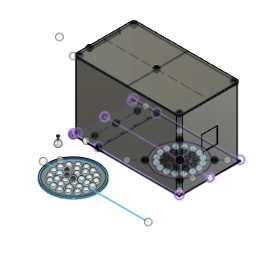
smallAmp v14 (Autodesk Fusion 360 design; units mm, degrees)
Autodesk Fusion 360 part; units mm, degrees
note: some values were not read from the file. Set by a fixed rule: which sketch regions a step uses.
sketch "Base" plane through (0, 0, 0) normal (0, 1, 0) x (1, 0, 0) in component "Top"
  line L0 (0, 0) -> (140, 0)
  line L1 (140, 0) -> (140, 80)
  line L2 (140, 80) -> (0, 80)
  line L3 (0, 80) -> (0, 0)
  dimension "d6" = 140
  dimension "d7" = 80
  constraint horizontal L0
  constraint vertical L1
  constraint horizontal L2
  constraint vertical L3
  constraint coincident L0.start L3.end
  measures "d6" distance of L0.start L0.end
  measures "d7" distance of L0.start L2.end
extrude "Extrude1" add sketch "Base" along normal blind 90 makes body 1 in component "Top"
fillet "Fillet1" radius 4 4 edges at (140, 45, 0) (0, 45, 0) (140, 45, -80) (0, 45, -80) on bodies 1 in component "Top"
shell "Shell1" thickness 1.5 removed faces 1 at (92, 90, -26.6667) on bodies 1 in component "Top"
sketch "Knob" plane through (1.5, 0, 0) normal (1, 0, 0) x (0, 0, -1) in component "Top"
  line L0 (76, 1.5) -> (76, 90)
  line L1 (76, 90) -> (4, 90)
  line L2 (4, 90) -> (4, 1.5)
  line L3 (4, 1.5) -> (76, 1.5)
  line L4 (20, 90) -> (60, 90)
  line L5 (60, 90) -> (60, 87)
  line L6 (60, 87) -> (20, 87)
  line L7 (20, 87) -> (20, 90)
  line L8 (40, 90) -> (40, 87) construction
  dimension "d12" = 40
  dimension "d13" = 3
  constraint horizontal L4
  constraint vertical L5
  constraint horizontal L6
  constraint vertical L7
  constraint coincident L1 L4.start
  constraint midpoint L1 L8.start
  constraint midpoint L6 L8.end
  constraint vertical L8
  measures "d12" distance of L5.end L6.end
  measures "d13" distance of L4.end L5.end
extrude "Extrude2" add sketch "Knob" along normal blind 6 draft -45 contours L1 L4 L5 L6 L7 bodies 1 in component "Top"
ref_plane "WorkPlane2" through (70, 45, -40) normal (-1, 0, 0) x (0, 0, 1) in component "Top"
mirror "Mirror1" about plane through (70, 45, -40) normal (-1, 0, 0) of "Extrude2" in component "Top"
sketch "Top" plane through (0, 90, 0) normal (0, 1, 0) x (-1, 0, 0) in component "Base"
  line L0 (-140, -4) -> (-140, -76)
  arc A0 (-140, -76) -> (-136, -80) centre (-136, -76) ccw
  line L1 (-136, -80) -> (-4, -80)
  arc A1 (-4, -80) -> (0, -76) centre (-4, -76) ccw
  line L2 (0, -76) -> (0, -4)
  arc A2 (0, -4) -> (-4, 0) centre (-4, -4) ccw
  line L3 (-4, 0) -> (-136, 0)
  arc A3 (-136, 0) -> (-140, -4) centre (-136, -4) ccw
  line L4 (-138.5, -20) -> (-138.5, -4)
  arc A4 (-136, -1.5) -> (-138.5, -4) centre (-136, -4) ccw
  line L5 (-136, -1.5) -> (-4, -1.5)
  arc A5 (-1.5, -4) -> (-4, -1.5) centre (-4, -4) ccw
  line L6 (-1.5, -4) -> (-1.5, -20)
  line L7 (-1.5, -20) -> (-1.5, -60)
  line L8 (-1.5, -60) -> (-1.5, -76)
  arc A6 (-4, -78.5) -> (-1.5, -76) centre (-4, -76) ccw
  line L9 (-4, -78.5) -> (-136, -78.5)
  arc A7 (-138.5, -76) -> (-136, -78.5) centre (-136, -76) ccw
  line L10 (-138.5, -76) -> (-138.5, -60)
  line L11 (-138.5, -60) -> (-138.5, -20)
  line L12 (0, -40) -> (-140, -40) construction
  line L13 (-70, -80) -> (-70, 0)
  point P0 (30.9232, -12.6835)
  point P1 (-70, -40)
  constraint midpoint L2 L12.start
  constraint midpoint L0 L12.end
  constraint midpoint L1 L13.start
  constraint midpoint L3 L13.end
  constraint midpoint L13 P1
extrude "Extrude1'" add sketch "Top" along normal blind 1.5 separate body makes body 2 in component "Base"
sketch "Lip" plane through (0, 90, 0) normal (0, -1, 0) x (1, 0, 0) in component "Base"
  arc A0 (140, -4) -> (136, 0) centre (136, -4) ccw
  line L0 (136, 0) -> (4, 0)
  arc A1 (4, 0) -> (0, -4) centre (4, -4) ccw
  line L1 (0, -4) -> (0, -76)
  arc A2 (0, -76) -> (4, -80) centre (4, -76) ccw
  line L2 (4, -80) -> (136, -80)
  arc A3 (136, -80) -> (140, -76) centre (136, -76) ccw
  line L3 (140, -76) -> (140, -4)
  line L4 (138.3, -76) -> (138.3, -4)
  arc A4 (138.3, -4) -> (136, -1.7) centre (136, -4) ccw
  line L5 (136, -1.7) -> (4, -1.7)
  arc A5 (4, -1.7) -> (1.7, -4) centre (4, -4) ccw
  line L6 (1.7, -4) -> (1.7, -76)
  arc A6 (1.7, -76) -> (4, -78.3) centre (4, -76) ccw
  line L7 (4, -78.3) -> (136, -78.3)
  arc A7 (136, -78.3) -> (138.3, -76) centre (136, -76) ccw
  dimension "d19" = 1.7
extrude "Extrude2'" add sketch "Lip" along normal blind 3 contours L4 A4 L5 A5 L6 A6 L7 A7 bodies 2 in component "Base"
extrude "Extrude3" cut sketch "Knob" along normal blind 3 draft -45 from surface at 0.2 contours L1 L4 L5 L6 L7 bodies 2 in component "Base"
mirror "Mirror1'" about plane through (70, 45, -40) normal (-1, 0, 0) of "Extrude3" in component "Base"
shell "Shell1'" thickness 1.5 removed faces 1 at (92.7667, 87, -46.6667) on bodies 2 in component "Base"
chamfer "Chamfer1" distance 0.6 angle 45 2 edges at (1.7, 87, -40) (138.3, 87, -40) on bodies 2 in component "Base"
ref_plane "WorkPlane1" through (70, 91.5, -40) normal (0, 1, 0) x (-1, 0, 0)
sketch "shelf" plane through (0, 1.5, 0) normal (0, 1, 0) x (-1, 0, 0)
  arc A0 (-4, -78.5) -> (-1.5, -76) centre (-4, -76) ccw
  line L0 (-1.5, -76) -> (-1.5, -4)
  arc A1 (-1.5, -4) -> (-4, -1.5) centre (-4, -4) ccw
  line L1 (-4, -1.5) -> (-136, -1.5)
  arc A2 (-136, -1.5) -> (-138.5, -4) centre (-136, -4) ccw
  line L2 (-138.5, -4) -> (-138.5, -76)
  arc A3 (-138.5, -76) -> (-136, -78.5) centre (-136, -76) ccw
  line L3 (-136, -78.5) -> (-4, -78.5)
  line L4 (-31.5, -78.5) -> (-33, -78.5)
  line L5 (-33, -78.5) -> (-33, -1.5)
  line L6 (-33, -1.5) -> (-31.5, -1.5)
  line L7 (-31.5, -1.5) -> (-31.5, -78.5)
  line L8 (-1.5, -76) -> (-1.5, -4)
  line L9 (-1.5, -40) -> (-140, -40) construction
  circle A4 centre (-100.5, -40) radius 28
  circle A5 centre (-100.5, -40) radius 29.5
  line L10 (-67.0739, -73.4261) -> (-135.1001, -5.3999) construction
  line L11 (-65.6316, -5.1316) -> (-131.9315, -71.4315) construction
  circle A6 centre (-77.519, -17.019) radius 1.25
  circle A7 centre (-77.519, -62.981) radius 1.25
  circle A8 centre (-123.481, -62.981) radius 1.25
  circle A9 centre (-123.481, -17.019) radius 1.25
  circle A10 centre (-77.519, -17.019) radius 2.5
  circle A11 centre (-77.519, -62.981) radius 2.5
  circle A12 centre (-123.481, -62.981) radius 2.5
  circle A13 centre (-123.481, -17.019) radius 2.5
  dimension "d121" = 30
  dimension "d122" = 1.5
  dimension "d125" = 56
  dimension "d126" = 38
  dimension "d127" = 1.5
  dimension "d130" = 45
  dimension "d131" = 45
  dimension "d132" = 2.5
  dimension "d133" = 32.5
  dimension "d134" = 2.5
  dimension "d135" = 2.5
  dimension "d136" = 2.5
  dimension "d137" = 32.5
  dimension "d138" = 32.5
  dimension "d139" = 32.5
  dimension "d140" = 5
  dimension "d141" = 5
  dimension "d142" = 5
  dimension "d143" = 5
  constraint horizontal L4
  constraint vertical L5
  constraint horizontal L6
  constraint vertical L7
  constraint coincident L1 L5.end
  constraint coincident L3 L4.start
  constraint midpoint L8 L9.start
  constraint perpendicular L2 L9
  constraint coincident L9 A4.centre
  constraint coincident A4.centre L10
  constraint coincident A4.centre L11
  constraint coincident L11 A6.centre
  constraint coincident L10 A7.centre
  constraint coincident L11 A8.centre
  constraint coincident L10 A9.centre
  constraint concentric A6 A10
  constraint concentric A7 A11
  constraint concentric A8 A12
  constraint concentric A9 A13
  measures "d121" distance of L7 L8
  measures "d122" distance of L5 L7
  measures "d125" diameter of A4
  measures "d126" distance of L2 A4.centre
  measures "d130" angle of L9 L10
  measures "d131" angle of L9 L11
  measures "d132" diameter of A6
  measures "d133" distance of A4.centre A6.centre
  measures "d134" diameter of A7
  measures "d135" diameter of A8
  measures "d136" diameter of A9
  measures "d137" distance of A4.centre A7.centre
  measures "d138" distance of A4.centre A8.centre
  measures "d139" distance of A4.centre A9.centre
  measures "d140" diameter of A10
  measures "d141" diameter of A11
  measures "d142" diameter of A12
  measures "d143" diameter of A13
extrude "Extrude5" add sketch "shelf" along normal blind 40 contours L1 L3 L4 L5 L6 L7 bodies 1 in component "Top"
extrude "Extrude6" add sketch "shelf" along normal blind 5 contours A5 bodies 1 in component "Top"
extrude "Extrude7" add sketch "shelf" along normal blind 5 contours A10 | A11 | A12 | A13 bodies 1 in component "Top"
sketch "connections" plane through (0, 1.5, 0) normal (0, 1, 0) x (-1, 0, 0)
  line L0 (-16.5, -0.6807) -> (-16.5, -79.3193) construction
  circle A0 centre (-16.5, -40) radius 3
  line L1 (-31.5, -1.5) -> (-31.5, -78.5) construction
  circle A1 centre (-16.5, -68) radius 2
  circle A2 centre (-16.5, -12) radius 2
  line L2 (-140, -80) -> (0, -80)
  line L3 (0, 0) -> (-140, 0)
  point P0 (-1.5, -40)
  dimension "d146" = 6
  dimension "d147" = 15
  dimension "d148" = 4
  dimension "d149" = 4
  dimension "d150" = 12
  dimension "d151" = 12
  constraint vertical L0
  constraint midpoint L0 A0.centre
  constraint horizontal A0.centre P0
  constraint coincident L0 A1.centre
  constraint coincident L0 A2.centre
  measures "d146" diameter of A0
  measures "d147" distance of L0 L1
  measures "d148" diameter of A1
  measures "d149" diameter of A2
  measures "d150" distance of A1.centre L2
  measures "d151" distance of A2.centre L3
extrude "Extrude8" cut sketch "connections" against normal through all bodies 1 in component "Top"
sketch "speakerholes" plane through (0, 1.5, 0) normal (0, 1, 0) x (-1, 0, 0)
  circle A0 centre (-118.6085, -27.5068) radius 2.5
  circle A1 centre (-100.5, -40) radius 27.32 construction
  circle A2 centre (-122.0111, -35.3876) radius 2.5
  circle A3 centre (-122.1387, -43.9706) radius 2.5
  circle A4 centre (-118.9721, -51.9491) radius 2.5
  circle A5 centre (-112.9932, -58.1085) radius 2.5
  circle A6 centre (-105.1124, -61.5111) radius 2.5
  circle A7 centre (-96.5294, -61.6387) radius 2.5
  circle A8 centre (-88.5509, -58.4721) radius 2.5
  circle A9 centre (-82.3915, -52.4932) radius 2.5
  circle A10 centre (-78.9889, -44.6124) radius 2.5
  circle A11 centre (-78.8613, -36.0294) radius 2.5
  circle A12 centre (-82.0279, -28.0509) radius 2.5
  circle A13 centre (-88.0068, -21.8915) radius 2.5
  circle A14 centre (-95.8876, -18.4889) radius 2.5
  circle A15 centre (-104.4706, -18.3613) radius 2.5
  circle A16 centre (-112.4491, -21.5279) radius 2.5
  line L0 (-100.5, -40) -> (-129.6267, -27.9353) construction
  line L1 (-1.5, -40) -> (-140, -40)
  circle A17 centre (-114.3582, -34.2597) radius 2.5
  circle A18 centre (-100.5, -40) radius 28
  circle A19 centre (-115.0855, -43.5017) radius 2.5
  circle A20 centre (-110.2417, -51.4061) radius 2.5
  circle A21 centre (-101.6769, -54.9538) radius 2.5
  circle A22 centre (-92.6625, -52.7896) radius 2.5
  circle A23 centre (-86.6418, -45.7403) radius 2.5
  circle A24 centre (-85.9145, -36.4983) radius 2.5
  circle A25 centre (-90.7583, -28.5939) radius 2.5
  circle A26 centre (-99.3231, -25.0462) radius 2.5
  circle A27 centre (-108.3375, -27.2104) radius 2.5
  circle A28 centre (-108.5, -40) radius 2.5
  circle A29 centre (-102.9721, -47.6085) radius 2.5
  circle A30 centre (-94.0279, -44.7023) radius 2.5
  circle A31 centre (-94.0279, -35.2977) radius 2.5
  circle A32 centre (-102.9721, -32.3915) radius 2.5
  circle A33 centre (-100.5, -40) radius 2.5
  point P0 (-100.5, -40)
  dimension "d154" = 5
  dimension "d156" = 360
  dimension "d157" = 22.5
  dimension "d158" = 5
  dimension "d159" = 22
  dimension "d160" = 15
  dimension "d162" = 360
  dimension "d163" = 5
  dimension "d164" = 8
  dimension "d166" = 360
  dimension "d167" = 5
  constraint coincident P0 A1.centre
  constraint coincident L0 A17.centre
  constraint coincident L1 A28.centre
  measures "d154" diameter of A0
  measures "d157" angle of L0 L1
  measures "d158" diameter of A17
  measures "d159" distance of A0.centre P0
  measures "d160" distance of P0 A17.centre
  measures "d163" diameter of A28
  measures "d164" distance of P0 A28.centre
  measures "d167" diameter of A33
extrude "Extrude9" cut sketch "speakerholes" against normal through all contours A0 | A2 | A3 | A4 | A5 | A6 | A7 | A8 | A9 | A10 | A11 | A12 | A13 | A14 | A15 | A16 | L1 A33 | L1 A33 | L1 A28 | L1 A28 | A17 | A19 | A20 | A21 | A22 | A23 | A24 | A25 | A26 | A27 | A29 | A30 | A31 | A32 bodies 1 in component "Top"
sketch "logoHole" plane through (140, 0, 0) normal (1, 0, 0) x (0, 0, -1)
  line L0 (76, 90) -> (4, 90)
  line L1 (4, 90) -> (4, 0)
  line L2 (4, 0) -> (76, 0)
  line L3 (76, 0) -> (76, 90)
  line L4 (4, 45) -> (76, 45) construction
  line L5 (40, 90) -> (40, 0) construction
  line L6 (50.5, 34.5) -> (29.5, 34.5)
  line L7 (29.5, 34.5) -> (29.5, 55.5)
  line L8 (29.5, 55.5) -> (50.5, 55.5)
  line L9 (50.5, 55.5) -> (50.5, 34.5)
  line L10 (50.5, 34.5) -> (29.5, 55.5) construction
  line L11 (29.5, 34.5) -> (50.5, 55.5) construction
  point P0 (40, 45)
  dimension "d169" = 21
  dimension "d170" = 21
  constraint midpoint L1 L4.start
  constraint midpoint L3 L4.end
  constraint midpoint L0 L5.start
  constraint midpoint L2 L5.end
  constraint horizontal L6
  constraint perpendicular L6 L7
  constraint parallel L6 L8
  constraint parallel L7 L9
  constraint coincident L10 P0
  constraint coincident L11 P0
  constraint midpoint L5 P0
  measures "d169" distance of L7.end L8.end
  measures "d170" distance of L6.end L7.end
extrude "Extrude10" cut sketch "logoHole" against normal blind 0.8 contours L6 L7 L8 L9 bodies 1 in component "Top"
sketch "ampstand" plane through (33, 0, 0) normal (1, 0, 0) x (0, 0, -1)
  line L0 (1.5, 1.5) -> (78.5, 1.5)
  line L1 (78.5, 1.5) -> (78.5, 41.5)
  line L2 (78.5, 41.5) -> (1.5, 41.5)
  line L3 (1.5, 41.5) -> (1.5, 1.5)
  circle A0 centre (16, 5) radius 2.5
  circle A1 centre (64, 5) radius 2.5
  circle A2 centre (64, 31) radius 2.5
  circle A3 centre (16, 31) radius 2.5
  circle A4 centre (16, 5) radius 1.4
  circle A5 centre (64, 5) radius 1.4
  circle A6 centre (64, 31) radius 1.4
  circle A7 centre (16, 31) radius 1.4
  line L4 (73.4261, 1.5) -> (5.3999, 1.5)
  line L5 (64, 5) -> (16, 5) construction
  point P0 (40, 5)
  point P1 (40, 1.5)
  dimension "d173" = 5
  dimension "d174" = 5
  dimension "d175" = 5
  dimension "d176" = 5
  dimension "d177" = 2.8
  dimension "d178" = 2.8
  dimension "d179" = 2.8
  dimension "d180" = 2.8
  dimension "d181" = 3.5
  dimension "d182" = 26
  dimension "d183" = 48
  dimension "d184" = 26
  constraint concentric A0 A4
  constraint concentric A1 A5
  constraint concentric A2 A6
  constraint concentric A3 A7
  constraint vertical A1.centre A2.centre
  constraint horizontal A3.centre A2.centre
  constraint coincident A1.centre A5.centre
  constraint coincident A0.centre A4.centre
  constraint midpoint L5 P0
  constraint vertical P0 P1
  constraint vertical A0.centre A3.centre
  measures "d173" diameter of A0
  measures "d174" diameter of A1
  measures "d175" diameter of A2
  measures "d176" diameter of A3
  measures "d177" diameter of A4
  measures "d178" diameter of A5
  measures "d179" diameter of A6
  measures "d180" diameter of A7
  measures "d181" distance of A0.centre L4
  measures "d182" vertical distance of A0.centre A3.centre
  measures "d183" horizontal distance of A0.centre A1.centre
  measures "d184" distance of A1.centre A2.centre
extrude "Extrude11" add sketch "ampstand" along normal blind 8 contours A0 | A1 | A2 | A3 bodies 1 in component "Top"
sketch "amphole" plane through (0, 1.5, 0) normal (0, 1, 0) x (-1, 0, 0)
  circle A0 centre (-49, -39.9687) radius 4.5
  line L0 (-33, -78.5) -> (-33, -1.5)
  dimension "d187" = 9
  dimension "d188" = 16
  measures "d187" diameter of A0
  measures "d188" distance of A0.centre L0
extrude "Extrude12" cut sketch "amphole" against normal through all bodies 1 in component "Top"
sketch "bezal" plane through (0, 0, 0) normal (0, 1, 0) x (1, 0, 0)
  circle A0 centre (0, -20) radius 2
  circle A1 centre (0, -20) radius 1.5
  dimension "d191" = 4
  dimension "d192" = 3
  constraint concentric A0 A1
  measures "d191" diameter of A0
  measures "d192" diameter of A1
extrude "Extrude1''" add sketch "bezal" against normal blind 1 separate body contours A0 | A1 makes body 3
extrude "Extrude2''" add sketch "bezal" along normal blind 9 contours A1 bodies 3
sketch "Sketch21" plane through (0, 0, 0) normal (0, 1, 0) x (1, 0, 0)
  circle A0 centre (50, -50) radius 32.5
  circle A1 centre (50, -50) radius 30.5
  circle A2 centre (49.9912, -50.0688) radius 27.32 construction
  line L0 (49.9912, -50.0688) -> (20.8645, -38.0042) construction
  circle A3 centre (46.0206, -28.4301) radius 2.5
  circle A4 centre (49.9912, -50.0688) radius 28
  circle A5 centre (49.9912, -50.0688) radius 2.5
  circle A6 centre (28.4802, -45.4564) radius 2.5
  circle A7 centre (71.5023, -54.6812) radius 2.5
  circle A8 centre (31.5191, -62.018) radius 2.5
  circle A9 centre (37.498, -68.1774) radius 2.5
  circle A10 centre (47.5191, -57.6773) radius 2.5
  circle A11 centre (54.6036, -28.5578) radius 2.5
  circle A12 centre (61.9404, -68.5409) radius 2.5
  circle A13 centre (45.3788, -71.5799) radius 2.5
  circle A14 centre (56.4633, -54.7711) radius 2.5
  circle A15 centre (57.8287, -62.8584) radius 2.5
  circle A16 centre (68.0997, -62.5621) radius 2.5
  circle A17 centre (59.7329, -38.6627) radius 2.5
  circle A18 centre (63.8494, -55.8091) radius 2.5
  circle A19 centre (35.4057, -53.5705) radius 2.5
  circle A20 centre (53.9618, -71.7076) radius 2.5
  circle A21 centre (28.3525, -54.0394) radius 2.5
  circle A22 centre (48.8143, -65.0226) radius 2.5
  circle A23 centre (68.4633, -38.1197) radius 2.5
  circle A24 centre (36.133, -44.3286) radius 2.5
  circle A25 centre (40.2495, -61.4749) radius 2.5
  circle A26 centre (47.5191, -42.4604) radius 2.5
  circle A27 centre (31.8827, -37.5756) radius 2.5
  circle A28 centre (38.0421, -31.5967) radius 2.5
  circle A29 centre (41.9912, -50.0688) radius 2.5
  circle A30 centre (56.4633, -45.3666) radius 2.5
  line L1 (148.9912, -50.0688) -> (10.4912, -50.0688)
  circle A31 centre (51.1681, -35.1151) radius 2.5
  circle A32 centre (42.1537, -37.2792) radius 2.5
  circle A33 centre (64.5768, -46.5672) radius 2.5
  circle A34 centre (71.6299, -46.0982) radius 2.5
  circle A35 centre (62.4845, -31.9603) radius 2.5
  point P0 (49.9912, -50.0688)
  dimension "d197" = 65
  dimension "d198" = -2
  dimension "d204" = 360
  dimension "d206" = 360
  dimension "d208" = 360
  dimension "d209" = 5
  dimension "d210" = 22.5
  dimension "d211" = 5
  dimension "d212" = 22
  dimension "d213" = 15
  dimension "d214" = 5
  dimension "d215" = 8
  dimension "d216" = 5
  constraint coincident P0 A2.centre
  constraint coincident A24.centre L0
  constraint coincident A29.centre L1
  measures "d197" diameter of A0
  measures "d209" diameter of A27
  measures "d210" angle of L0 L1
  measures "d211" diameter of A24
  measures "d212" distance of P0 A27.centre
  measures "d213" distance of A24.centre P0
  measures "d214" diameter of A29
  measures "d215" distance of A29.centre P0
  measures "d216" diameter of A5
extrude "Extrude3'" add sketch "Sketch21" along normal blind 1 separate body contours A0 A1 L1 | A0 A1 L1 | A1 A4 L1 | A1 A4 L1 | A4 A5 A29 L1 | A4 A5 A29 L1 | A29 L1 | A29 L1 | A5 L1 | A5 L1 | A3 | A6 | A7 | A8 | A9 | A10 | A11 | A12 | A13 | A14 | A15 | A16 | A17 | A18 | A19 | A20 | A21 | A22 | A23 | A24 | A25 | A26 | A27 | A28 | A30 | A31 | A32 | A33 | A34 | A35 makes body 4
extrude "Extrude4" add sketch "Sketch21" along normal blind 2 contours A0 A1 L1 | A0 A1 L1 bodies 4
extrude "Extrude5'" cut sketch "Sketch21" along normal through all contours A29 L1 | A29 L1 | A5 L1 | A5 L1 | A3 | A6 | A7 | A8 | A9 | A10 | A11 | A12 | A13 | A14 | A15 | A16 | A17 | A18 | A19 | A20 | A21 | A22 | A23 | A24 | A25 | A26 | A27 | A28 | A30 | A31 | A32 | A33 | A34 | A35 bodies 4
component "Enclosure" placed x (1, 0, 0) y (0, 1, 0) z (0, 0, 1) at (0, 0, 0)
component "Top" placed x (1, 0, 0) y (0, 1, 0) z (0, 0, 1) at (0, 0, 0) in component "Enclosure"
component "Base" placed x (1, 0, 0) y (0, 1, 0) z (0, 0, 1) at (0, 0, 0) in component "Enclosure"
equation "Width = 80 mm"
equation "length = 140 mm"
equation "heigth = 90 mm"
equation "shell = 1.5 mm"
equation "gap = 0.2 mm"
equation "d6 = length"
equation "d7 = Width"
equation "d8 = heigth"
equation "d11 = shell"
equation "d12 = Width / 2"
equation "d13 = shell * 2"
equation "d17 = shell"
equation "d19 = shell + gap"
equation "d20 = shell * 2"
equation "d23 = shell * 2"
equation "d26 = shell"
equation "d122 = shell"
equation "d126 = 56 mm / 2 + 10 mm"
equation "d127 = shell"
equation "d133 = ( 65 / 2 ) * 1 mm"
equation "d137 = ( 65 / 2 ) * 1 mm"
equation "d138 = ( 65 / 2 ) * 1 mm"
equation "d139 = ( 65 / 2 ) * 1 mm"
equation "d157 = ( 45 / 2 ) * 1 deg"
equation "d210 = ( 45 / 2 ) * 1 deg"
